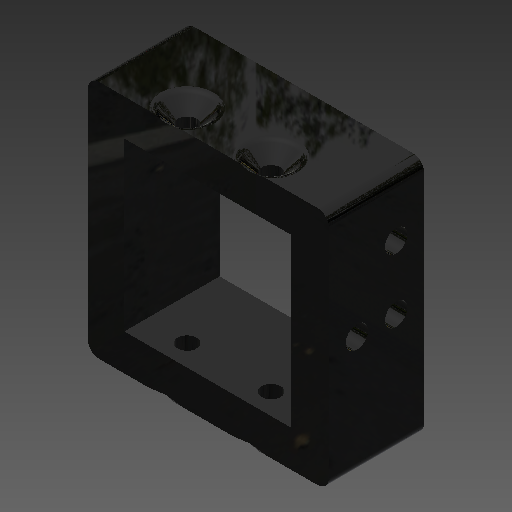
# Autodesk Inventor part: 3d_JacintoDevKit_Addon - Panel bracket
Saved by Autodesk Inventor 2018.3 (Build 223284000, 284)
## iProperties
Category: 0
Created: 2025-11-24
Part Number: 3d_JacintoDevKit_Addon - Panel bracket
Material: PA12 SLS 3D Print
Document SubType Name: Modeling
Designer: mbs18
Density: 0.95 g/cm^3
Appearance: Black
Manufacturer-1: {"Link": "", "Name": "TECNOBRO 3D SL", "PartNumber": "3d_JacintoDevKit_Addon - Panel bracket", "partner_id": false}
Manufacturer-2: {"Link": "", "Name": "", "PartNumber": "", "partner_id": false}
Manufacturer-3: {"Link": "", "Name": "", "PartNumber": "", "partner_id": false}
Manufacturer-4: {"Link": "", "Name": "", "PartNumber": "", "partner_id": false}
Manufacturer-5: {"Link": "", "Name": "", "PartNumber": "", "partner_id": false}
Provider-1: {"Link": "", "Name": "", "PartNumber": "", "partner_id": false}
Provider-2: {"Link": "", "Name": "", "PartNumber": "", "partner_id": false}
Provider-3: {"Link": "", "Name": "", "PartNumber": "", "partner_id": false}
Provider-4: {"Link": "", "Name": "", "PartNumber": "", "partner_id": false}
Provider-5: {"Link": "", "Name": "", "PartNumber": "", "partner_id": false}
odoo_id: 22002
odoo_internal_code: P014367
odoo_model: product.product
odoo_x2o_application_version: 12.0.4.20
odoo_d2o_version: 12.0.1.6.0
Author: mbs18
Comments: DIN-ISO-2768-mK
Autodesk Inventor part; units mm, degrees
ref_plane "YZ Plane" through (0, 0, 0) normal (1, 0, 0) x (0, 1, 0)
ref_plane "XZ Plane" through (0, 0, 0) normal (0, 1, 0) x (-1, 0, 0)
sketch "Sketch7" plane through (0, 0, 0) normal (0, 0, 1) x (1, 0, 0)
  line L0 (0, 0) -> (14.8, 0)
  line L1 (14.8, 0) -> (14.8, 14.8)
  line L2 (14.8, 14.8) -> (14.8, -15)
  line L3 (14.8, -15) -> (17.8, -15)
  line L4 (17.8, -15) -> (17.8, 21.3)
  line L5 (14.8, 14.8) -> (-15, 14.8)
  line L6 (14.8, 14.8) -> (44.6, 14.8) construction
  line L7 (-15, 14.8) -> (-15, -15)
  line L8 (-15, -15) -> (-18, -15)
  line L9 (-18, -15) -> (-18, 21.3)
  line L10 (-18, 21.3) -> (17.8, 21.3)
  dimension "d54" = 14.8
  dimension "d55" = 14.8
  dimension "d56" = 90
  dimension "d57" = 29.8
  dimension "d58" = 3
  dimension "d60" = 29.8
  dimension "d61" = 180
  dimension "d62" = 29.8
  dimension "d63" = 90
  dimension "d64" = 3
  dimension "d129" = 36.3
  constraints: 22 end point, 8 perpendicular, 2 horizontal, 1 collinear, 1 point on line
  measures "d54" distance of L0.start L0.end
  measures "d55" distance of L0.end L1.end
  measures "d56" angle of L1 L0
  measures "d57" distance of L1.end L2.end
  measures "d58" distance of L2.end L3.end
  measures "d60" distance of L1.end L5.end
  measures "d61" angle of L5 L6
  measures "d62" distance of L5.end L7.end
  measures "d63" angle of L7 L5
  measures "d64" distance of L7.end L8.end
  measures "d129" distance between parallel lines of L10 L3
extrude "Extrusion7" add sketch "Sketch7" against normal blind 24
sketch "Sketch8" plane through (17.8, -15, 0) normal (1, 0, 0) x (0, 0, -1)
  line L0 (0, 0) -> (0, 36.3) projected
  point P0 (0, 15)
  point P1 (4, 22.4)
  point P2 (4, 7.4)
  point P3 (0, 29.8)
  dimension "d68" = 15
  dimension "d69" = 4
  dimension "d70" = 7.4
  constraints: 1 vertical alignment
  measures "d68" distance of point (4, 7.4) point (4, 22.4)
  measures "d69" distance from line of point (4, 22.4) L0
  measures "d70" vertical distance of point (4, 22.4) point (0, 29.8)
hole "Hole1" at (17.8, 7.4, -4) at (17.8, -7.6, -4) direction (-1, 0, 0) diameter 3.4 end through all
sketch "Sketch9" plane through (17.8, -15, 0) normal (1, 0, 0) x (0, 0, -1)
  circle A0 centre (12, 14.9) radius 21 construction
  line L0 (0, 36.3) -> (24, 36.3) projected
  circle A1 centre (4, 22.4) radius 1.7 projected
  circle A2 centre (4, 7.4) radius 1.7 projected
  line L1 (4, 22.4) -> (4, 7.4) construction
  circle A3 centre (12, 14.9) radius 5 construction
  line L2 (0, 0) -> (24, 0) construction
  line L3 (0, 0) -> (10, 0) construction
  line L4 (10, 0) -> (16.4522, 12.6245)
  line L5 (17, 14.9) -> (17, 36.3)
  arc A4 (16.4522, 12.6245) -> (17, 14.9) centre (12, 14.9) ccw
  line L6 (10, 0) -> (24, 0)
  line L7 (24, 0) -> (24, 36.3)
  line L8 (24, 0) -> (24, 29.8) projected
  line L9 (17, 36.3) -> (24, 36.3)
  point P0 (0, 15)
  point P1 (12, 36.3)
  point P2 (4, 14.9)
  dimension "d78" = 42
  dimension "d79" = 10
  dimension "d80" = 10
  constraints: 14 end point, 4 point on circle, 3 centre point, 2 coincident, 2 collinear, 2 midpoint, 2 point on line, 2 tangent, 1 concentric, 1 horizontal, 1 horizontal alignment, 1 perpendicular, 1 vertical, 1 vertical alignment
  measures "d78" diameter of A0
  measures "d79" diameter of A3
  measures "d80" distance of L2.start L3.end
extrude "Extrusion8" cut sketch "Sketch9" against normal up to next contours L0 L7 L6 L4 A4 L5
sketch "Sketch10" plane through (17.8, -0.1, -17) normal (1, 0, 0) x (0, 0, -1)
  arc A0 (-0.5478, -2.2755) -> (0, 0) centre (-5, 0) ccw projected
  circle A1 centre (-5, 0) radius 6
  point P0 (-17, 0.1)
  dimension "d84" = 12
  constraints: 1 centre point, 1 coincident
  measures "d84" diameter of A1
extrude "Extrusion9" add sketch "Sketch10" along normal blind 3.7
mirror "Mirror2" about plane through (0, 0, 0) normal (1, 0, 0) of "Extrusion9"
sketch "Sketch12" plane through (21.5, -0.1, -12) normal (1, 0, 0) x (0, 0, -1)
  circle A0 centre (0, 0) radius 6 projected
  point P0 (-12, 0.1)
  point P1 (0, 0)
  constraints: 1 coincident
hole "Hole2" at (21.5, -0.1, -12) direction (-1, 0, 0) diameter 4 depth 5.7
mirror "Mirror3" about plane through (0, 0, 0) normal (1, 0, 0) of "Hole2"
sketch "Sketch13" plane through (17.8, -0.1, -17) normal (-1, 0, 0) x (0, 0, 1)
  line L0 (0, 0) -> (0, 3.3166) projected
  arc A0 (0, 3.3166) -> (2.0572, -5.2287) centre (5, 0) ccw projected
  line L1 (2.0572, -5.2287) -> (0.5478, -2.2755) projected
  arc A1 (0, 0) -> (0.5478, -2.2755) centre (5, 0) ccw projected
  point P0 (17, 0.1)
extrude "Extrusion11" cut sketch "Sketch13" along normal mid plane 111.5
sketch "Sketch15" plane through (17.8, 21.3, 0) normal (1, 0, 0) x (0, 0, -1)
  arc A0 (17, -18.0834) -> (14.9428, -26.6287) centre (12, -21.4) ccw projected
  line L0 (17, -18.0834) -> (17, 0) projected
  line L1 (0, 0) -> (17, 0) projected
  line L2 (0, -36.3) -> (0, 0) projected
  line L3 (0, -36.3) -> (10, -36.3) projected
  line L4 (10, -36.3) -> (14.9428, -26.6287) projected
  circle A1 centre (4, -13.9) radius 1.7 projected
  circle A2 centre (4, -28.9) radius 1.7 projected
  point P0 (0, -21.3)
extrude "Extrusion12" add sketch "Sketch15" along normal up to surface (3.7 mm away)
sketch "Sketch16" plane through (-18, 21.3, -17) normal (-1, 0, 0) x (0, 0, 1)
  arc A0 (2.0572, -26.6287) -> (0, -18.0834) centre (5, -21.4) ccw projected
  line L0 (2.0572, -26.6287) -> (7, -36.3) projected
  line L1 (17, -36.3) -> (7, -36.3) projected
  line L2 (17, 0) -> (17, -36.3) projected
  line L3 (17, 0) -> (0, 0) projected
  line L4 (0, 0) -> (0, -18.0834) projected
  circle A1 centre (13, -13.9) radius 1.7 projected
  circle A2 centre (13, -28.9) radius 1.7 projected
  point P0 (17, -21.3)
extrude "Extrusion13" add sketch "Sketch16" along normal up to surface (3.5 mm away)
fillet "Fillet8" radius 2 2 edges at (-21.5, 21.3, -8.5) (21.5, 21.3, -8.5)
sketch "Sketch17" plane through (21.5, -0.1, -17) normal (1, 0, 0) x (0, 0, -1)
  line L0 (-7, -14.9) -> (-0.5478, -2.2755) projected
  line L1 (-17, -21.4) -> (-17, -14.9)
  line L2 (-17, -14.9) -> (-7, -14.9) projected
  line L3 (-17, -14.9) -> (-7, -14.9)
  line L4 (0, 0) -> (0, 19.4) projected
  line L5 (0, 0) -> (0, -21.4)
  line L6 (0, -21.4) -> (-17, -21.4)
  arc A0 (-0.5478, -2.2755) -> (0, 0) centre (-5, 0) ccw projected
  line L7 (-7, -14.9) -> (-0.5478, -2.2755)
  arc A1 (-0.5478, -2.2755) -> (0, 0) centre (-5, 0) ccw
  point P0 (-17, 0.1)
  point P1 (-17, -14.9)
  dimension "d145" = 6.5
  dimension "d146" = 17
  constraints: 10 end point, 2 horizontal, 2 point on circle, 1 centre point, 1 coincident, 1 tangent, 1 vertical
  measures "d145" distance of L1.start L1.end
  measures "d146" distance of L5.end L1.start
extrude "Extrusion14" add sketch "Sketch17" against normal up to surface (6.7 mm away)
sketch "Sketch19" plane through (-21.5, -15, -10) normal (-1, 0, 0) x (0, 0, 1)
  line L0 (10, 0) -> (10, 29.8) projected
  line L1 (10, 29.8) -> (10, -6.5) projected
  line L2 (10, 0) -> (10, -6.5)
  line L3 (-7, 29.8) -> (-7, -6.5) projected
  line L4 (10, -6.5) -> (-7, -6.5)
  arc A0 (-7, 14.9) -> (-6.4522, 12.6245) centre (-2, 14.9) ccw projected
  line L5 (-7, -6.5) -> (-7, 14.9)
  line L6 (10, 0) -> (0, 0) projected
  line L7 (10, 0) -> (0, 0)
  line L8 (-6.4522, 12.6245) -> (0, 0) projected
  line L9 (0, 0) -> (-6.4522, 12.6245)
  arc A1 (-7, 14.9) -> (-6.4522, 12.6245) centre (-2, 14.9) ccw
  point P0 (10, 15)
  constraints: 10 end point, 3 collinear, 2 perpendicular, 2 point on circle, 2 tangent, 1 centre point, 1 concentric
extrude "Extrusion15" add sketch "Sketch19" against normal up to surface (6.5 mm away)
sketch "Sketch20" plane through (14.8, 14.8, -17) normal (-1, 0, 0) x (0, 0, 1)
  line L0 (17, -36.3) -> (0, -36.3) projected
  line L1 (0, -36.3) -> (0, 4.5) projected
  line L2 (17, -36.3) -> (0, -36.3)
  line L3 (0, -36.3) -> (0, -29.8)
  line L4 (0, -29.8) -> (17, -29.8)
  line L5 (17, -29.8) -> (17, -36.3)
  point P0 (17, -14.8)
  dimension "d149" = 6.5
  constraints: 8 end point, 2 parallel, 1 horizontal, 1 perpendicular, 1 point on line
  measures "d149" distance of L2.end L3.end
extrude "Extrusion16" add sketch "Sketch20" along normal up to surface (29.8 mm away)
fillet "Fillet11" radius 2 2 edges at (-21.5, -21.5, -8.5) (21.5, -21.5, -8.5)
ref_plane "Work Plane1" through (14.65, -13.7878, -25.4761) normal (1, 0, 0) x (0, 1, 0)
sketch "Sketch21" plane through (21.5, -0.1, -17) normal (1, 0, 0) x (0, 0, -1)
  circle A0 centre (-13, 7.5) radius 1.7 projected
  circle A1 centre (-13, -7.5) radius 1.7 projected
  point P0 (-17, 0.1)
extrude "Extrusion17" add sketch "Sketch21" against normal blind 6.7
sketch "Sketch22" plane through (-19.5, 21.3, -17) normal (0, 1, 0) x (1, 0, 0)
  circle A0 centre (11.9, -13.2) radius 1.2295 projected
  circle A1 centre (26.9, -13.2) radius 1.2295 projected
  point P0 (19.5, -17)
sketch "Sketch23" plane through (-21.5, 19.3, -17) normal (-1, 0, 0) x (0, 0, 1)
  circle A0 centre (13, -11.9) radius 1.7 projected
  circle A1 centre (13, -26.9) radius 1.7 projected
  point P0 (17, -19.3)
extrude "Extrusion18" add sketch "Sketch23" against normal blind 6.5
hole "Hole4" at (-7.6, 21.3, -3.8) at (7.4, 21.3, -3.8) direction (0, -1, 0) diameter 3.4 end through all
chamfer "Chamfer4" distance 2.5 angle 45 4 edges at (-7.6, 21.3, -5.5) (7.4, 21.3, -5.5) (7.4, -21.5, -5.5) (-7.6, -21.5, -5.5)
fillet "Fillet12" radius 1.5 4 edges at (-7.6, 21.3, -8) (7.4, 21.3, -8) (7.4, -21.5, -8) (-7.6, -21.5, -8)
sketch "Sketch27" plane through (-21.5, 19.3, -17) normal (-1, 0, 0) x (0, 0, 1)
  line L0 (17, 2) -> (0, 2) projected
  line L1 (0, 0) -> (0, -38.8) projected
  circle A0 centre (-6.3513, -19.4) radius 1.85 projected
  circle A1 centre (5, -19.4) radius 2 projected
  point P0 (17, -19.3)
  point P1 (5, -8.049)
  dimension "d186" = 10.049
  constraints: 1 vertical alignment
  measures "d186" distance from line of L0 point (5, -8.049)
hole "Hole5" at (-21.5, 11.251, -12) direction (1, 0, 0) diameter 4 depth 5.7
sketch "Sketch28" plane through (21.5, -0.1, -17) normal (1, 0, 0) x (0, 0, -1)
  circle A0 centre (-5, 11.351) radius 1.2295 projected
  point P0 (-17, 0.1)
hole "Hole6" at (21.5, 11.251, -12) direction (-1, 0, 0) diameter 4 depth 5.7
sketch "Sketch29" plane through (21.5, -0.1, -17) normal (1, 0, 0) x (0, 0, -1)
  circle A0 centre (-11, 0) radius 1.85 projected
  point P0 (-17, 0.1)
  point P1 (-12, 0)
  dimension "d209" = 1
  constraints: 1 horizontal alignment
  measures "d209" distance of A0.centre point (-12, 0)
hole "Hole7" at (21.5, -0.1, -5) direction (-1, 0, 0) diameter 4 depth 5.7
sketch "Sketch30" plane through (-21.5, 19.3, -17) normal (-1, 0, 0) x (0, 0, 1)
  circle A0 centre (11, -19.4) radius 1.85 projected
  point P0 (17, -19.3)
  point P1 (12, -19.4)
  dimension "d208" = 1
  constraints: 1 horizontal alignment
  measures "d208" distance of A0.centre point (12, -19.4)
hole "Hole8" at (-21.5, -0.1, -5) direction (1, 0, 0) diameter 4 depth 5.7
body "Solid2"
